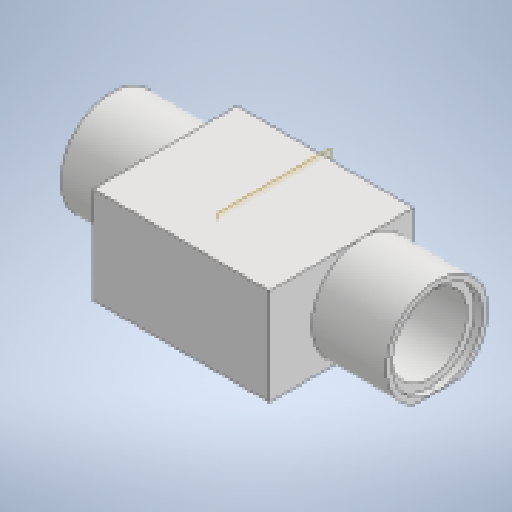
# Autodesk Inventor part: motors_mount
Saved by Autodesk Inventor 2023 (Build 270158000, 158)
## iProperties
Created: 2025-01-11
Part Number: motors_mount
Material: Ogólny
Document SubType Name: Modeling
Designer: kamil
Density: 1 g/cm^3
Appearance: Domyślna
Author: kamil
Autodesk Inventor part; units mm, degrees
ref_plane "YZ Plane" through (0, 0, 0) normal (1, 0, 0) x (0, 1, 0)
ref_plane "XZ Plane" through (0, 0, 0) normal (0, 1, 0) x (-1, 0, 0)
ref_plane "XY Plane" through (0, 0, 0) normal (0, 0, 1) x (1, 0, 0)
sketch "Szkic1" plane through (0, 0, 0) normal (1, 0, 0) x (0, 1, 0)
  circle A0 centre (0, 0) radius 11
  dimension "d0" = 22
  constraints: 1 centre point, 1 coincident
  measures "d0" diameter of A0
extrude "Wyciągnięcie proste1" add sketch "Szkic1" along normal blind 70
sketch "Szkic2" plane through (70, 0, 0) normal (1, 0, 0) x (0, 0, -1)
  circle A0 centre (0, 0) radius 11 projected
  circle A1 centre (0, 0) radius 9.75
  dimension "d3" = 19.5
  constraints: 1 centre point, 1 coincident
  measures "d3" diameter of A1
extrude "Wyciągnięcie proste2" cut sketch "Szkic2" against normal blind 1.6 contours A1
sketch "Szkic3" plane through (68.4, 0, 0) normal (1, 0, 0) x (0, 0, -1)
  circle A0 centre (0, 0) radius 9.75 projected
  circle A1 centre (0, 0) radius 8.15
  dimension "d6" = 16.3
  constraints: 1 centre point, 1 coincident
  measures "d6" diameter of A1
extrude "Wyciągnięcie proste3" cut sketch "Szkic3" against normal blind 31 contours A1
ref_plane "Płaszczyzna konstrukcyjna1" through (35, 0, 0) normal (1, 0, 0) x (0, 0, -1)
mirror "Odbij1" about plane through (35, 0, 0) normal (1, 0, 0) of "Wyciągnięcie proste3", "Wyciągnięcie proste2"
sketch "Szkic4" plane through (70, 0, 0) normal (1, 0, 0) x (0, 0, -1)
  circle A0 centre (0, 0) radius 11 projected
  line L0 (-20, 11) -> (11, 11)
  line L1 (11, 11) -> (11, -11)
  line L2 (11, -11) -> (-20, -11)
  line L3 (-20, -11) -> (-20, 11)
  point P0 (0, -11)
  point P1 (0, 11)
  dimension "d9" = 20
  constraints: 8 end point, 3 tangent, 2 parallel, 1 horizontal, 1 perpendicular
  measures "d9" distance from line of L3 point (0, 0)
extrude "Wyciągnięcie proste4" add sketch "Szkic4" against normal up to surface (70 mm away) contours A0 L2 L3 L0
sketch "Szkic5" plane through (70, 11, 20) normal (0, 1, 0) x (1, 0, 0)
  line L0 (-70, 0) -> (-70, 20) projected
  line L1 (-70, 31) -> (0, 31) projected
  line L2 (-37.4, 28.15) -> (-37.4, 11.85) projected
  line L3 (-68.4, 11.85) -> (-68.4, 28.15) projected
  line L4 (-37.4, 28.15) -> (-37.4, 11.85) projected
  line L5 (-37.4, 28.15) -> (-68.4, 28.15)
  line L6 (-37.4, 28.15) -> (-68.4, 28.15) projected
  line L7 (-68.4, 11.85) -> (-37.4, 11.85)
  line L8 (-70, 10.25) -> (-70, 29.75) projected
  line L9 (0, 0) -> (-70, 0) projected
  line L10 (-70, 0) -> (-54, 0)
  line L11 (-54, 0) -> (-54, 9)
  line L12 (-54, 9) -> (-70, 9)
  line L13 (-70, 9) -> (-70, 0)
  line L14 (0, 0) -> (-16, 0)
  line L15 (-16, 0) -> (-16, 9)
  line L16 (-16, 9) -> (0, 9)
  line L17 (0, 9) -> (0, 0)
  point P0 (-16, 0)
  dimension "d12" = 16
  dimension "d13" = 2.85
  dimension "d14" = 16
  constraints: 20 end point, 5 equal length, 3 perpendicular, 2 horizontal
  measures "d12" distance of L12.end L11.end
  measures "d13" distance between parallel lines of L7 L12
  measures "d14" distance of L15.end L16.end
extrude "Wyciągnięcie proste5" cut sketch "Szkic5" along normal through all both and the other way through all contours L0 L12 L11 L9 | L9 L15 L16 L17
sketch "Szkic6" plane through (0, 0, 0) normal (-1, 0, 0) x (0, 0, 1)
  arc A0 (0, 11) -> (0, -11) centre (0, 0) ccw projected
  circle A1 centre (0, 0) radius 11
  line L0 (11, -11) -> (11, 11) projected
  line L1 (11, 11) -> (0, 11) projected
  arc A2 (0, 11) -> (0, -11) centre (0, 0) ccw projected
  line L2 (0, -11) -> (11, -11) projected
  circle A3 centre (0, 0) radius 9.75 projected
  point P0 (0, -11)
  point P1 (11, 0)
  constraints: 1 coincident, 3 other
extrude "Wyciągnięcie proste6" cut sketch "Szkic6" against normal up to surface (16 mm away) contours L1 L0 A1 | A1 L0 L2
mirror "Odbij2" about plane through (35, 0, 0) normal (1, 0, 0) of "Wyciągnięcie proste6"
sketch "Szkic7" plane through (70, 0, 0) normal (1, 0, 0) x (0, 0, -1)
  line L0 (0, -11) -> (-20, -11) projected
  circle A0 centre (0, 0) radius 9.75 projected
  line L1 (-20, -11) -> (0, -11) projected
  line L2 (-20, -11) -> (9.75, -11)
  line L3 (9.75, -11) -> (9.75, -9.75)
  line L4 (9.75, -9.75) -> (-20, -9.75)
  line L5 (-20, -9.75) -> (-20, -11)
  constraints: 8 end point, 2 parallel, 2 tangent, 1 horizontal, 1 perpendicular
extrude "Wyciągnięcie proste7" cut sketch "Szkic7" against normal through all contours L0 L5 L4 L3 L2
sketch "Szkic8" plane through (54, 11, 20) normal (1, 0, 0) x (0, 0, -1)
  arc A0 (25.0929, -20.75) -> (14.9071, -20.75) centre (20, -11) ccw projected
  line L0 (0, -20.75) -> (14.9071, -20.75) projected
  line L1 (20, 0) -> (0, 0) projected
  line L2 (20, 0) -> (31, 0)
  line L3 (31, 0) -> (31, -20.75)
  line L4 (31, -20.75) -> (20, -20.75)
  line L5 (20, -20.75) -> (20, 0)
  point P0 (31, -11)
  constraints: 8 end point, 2 parallel, 1 collinear, 1 horizontal, 1 perpendicular, 1 tangent
extrude "Wyciągnięcie proste8" add sketch "Szkic8" against normal up to surface (38 mm away) contours A0 L3 L4 | A0 L2 L3
sketch "Szkic9" plane through (16, 11, 20) normal (0, 0, 1) x (1, 0, 0)
  line L0 (0, -20.75) -> (38, -20.75) projected
  line L1 (38, -20.75) -> (38, 0) projected
  line L2 (38, 0) -> (0, 0) projected
  line L3 (0, 0) -> (0, -20.75) projected
  point P0 (-16, -11)
extrude "Wyciągnięcie proste9" cut sketch "Szkic9" against normal blind 3
sketch "Szkic10" plane through (54, 11, 0) normal (0, 1, 0) x (1, 0, 0)
  line L0 (-38, -17) -> (0, -17) projected
  line L1 (0, -17) -> (0, 0) projected
  line L2 (0, 11) -> (0, 0) projected
  line L3 (0, 11) -> (-38, 11) projected
  line L4 (-38, 0) -> (-38, 11) projected
  line L5 (-38, 0) -> (-38, -17) projected
  point P0 (-54, 0)
  point P1 (-10, -13)
  point P2 (-28, -13)
  point P3 (-19, 5.5)
  point P4 (-19, 11)
  dimension "d26" = 10
  dimension "d27" = 4
  dimension "d28" = 10
  dimension "d29" = 4
  dimension "d30" = 5.5
  constraints: 1 midpoint, 1 vertical alignment
  measures "d26" distance from line of L1 point (-10, -13)
  measures "d27" distance from line of L0 point (-10, -13)
  measures "d28" distance from line of L5 point (-28, -13)
  measures "d29" distance from line of point (-28, -13) L0
  measures "d30" distance from line of L3 point (-19, 5.5)
hole "Otwór1" at (44, 11, 13) at (26, 11, 13) at (35, 11, -5.5) direction (0, -1, 0) diameter 3.4 end through all
sketch "Szkic11" plane through (54, 11, 0) normal (0, 1, 0) x (1, 0, 0)
  circle A0 centre (-19, 5.5) radius 1.7 projected
  circle A1 centre (-19, 5.5) radius 2.8
  line L0 (0, 11) -> (-38, 11) projected
  line L1 (0, 11) -> (-38, 11) projected
  line L2 (-21.8, 5.5) -> (-16.2, 5.5)
  line L3 (-16.2, 5.5) -> (-16.2, 11)
  line L4 (-16.2, 11) -> (-21.8, 11)
  line L5 (-21.8, 11) -> (-21.8, 5.5)
  point P0 (-54, 0)
  dimension "d38" = 1.1
  constraints: 8 end point, 2 parallel, 2 vertical, 1 horizontal, 1 perpendicular, 1 point on line, 3 other
extrude "Wyciągnięcie proste10" add sketch "Szkic11" against normal up to surface (20.75 mm away) contours L2 A1 A0 | A0 L2 A1 | A1 L5 L0 L3
chamfer "Faza1" distance 1 angle 45 1 edges at (35, -9.75, -11)
sketch "Szkic12" plane through (68.4, 0, 0) normal (1, 0, 0) x (0, 0, -1)
  circle A0 centre (0, 0) radius 9.75 projected
  line L0 (0, 0) -> (-6.2672, 7.4689)
  circle A1 centre (0, 0) radius 9.75 projected
  line L1 (0, 0) -> (9.75, 0) construction
  line L2 (-6.2672, 7.4689) -> (-5.0415, 8.4974)
  line L3 (-5.0415, 8.4974) -> (1.6116, 0.5686)
  line L4 (-6.2672, 7.4689) -> (-7.4929, 6.4405)
  line L5 (-7.4929, 6.4405) -> (-3.3968, 1.559)
  circle A2 centre (0, 0) radius 8.15 projected
  point P0 (0, -9.75)
  point P1 (-6.3624, 5.0933)
  point P2 (-3.9111, 7.1502)
  point P3 (-4.9565, 8.3961)
  point P4 (-7.4079, 6.3392)
  dimension "d44" = 130
  dimension "d45" = 1.6
  dimension "d46" = 1.6
  constraints: 12 end point, 1 collinear, 1 equal length, 1 horizontal, 1 parallel, 1 perpendicular, 1 point on circle, 1 tangent, 2 other
  measures "d44" angle of L1 L0
  measures "d45" distance of L0.end L2.end
  measures "d46" distance between parallel lines of L0 L5
extrude "Wyciągnięcie proste11" cut sketch "Szkic12" against normal up to surface (31 mm away) contours L3 A2 L0 A0 | A0 L0 A2 L5
sketch "Szkic13" plane through (16, 11, 17) normal (0, 0, 1) x (1, 0, 0)
  line L0 (38, 0) -> (38, -20.75) projected
  line L1 (0, 0) -> (38, 0) projected
  line L2 (0, -20.75) -> (0, 0) projected
  line L3 (38, -20.75) -> (0, -20.75) projected
  line L4 (21.4, -2.6039) -> (24.4, -2.6039)
  line L5 (24.4, -2.6039) -> (24.4, -4.6608)
  line L6 (24.4, -4.6608) -> (21.4, -4.6608)
  line L7 (21.4, -4.6608) -> (21.4, -2.6039)
  point P0 (-16, -11)
  dimension "d49" = 3
  constraints: 8 end point, 2 parallel, 1 coincident, 1 horizontal, 1 perpendicular
  measures "d49" distance of L5.end L6.end
extrude "Wyciągnięcie proste12" cut sketch "Szkic13" against normal up to surface (12.0435 mm away) contours L4 L5 L6 L7
sketch "Szkic14" plane through (37.4, 0, 0) normal (1, 0, 0) x (0, 0, -1)
  line L0 (-6.3624, 5.0933) -> (-7.4079, 6.3392) projected
  arc A0 (-6.3624, 5.0933) -> (4.0578, -7.068) centre (0, 0) ccw projected
  line L1 (4.0578, -7.068) -> (4.0578, 7.068) projected
  arc A1 (4.0578, 7.068) -> (-3.9111, 7.1502) centre (0, 0) ccw projected
  line L2 (-4.9565, 8.3961) -> (-3.9111, 7.1502) projected
  line L3 (-17, 8.3961) -> (-4.9565, 8.3961) projected
  line L4 (-17, 6.3392) -> (-17, 8.3961) projected
  line L5 (-17, 6.3392) -> (-7.4079, 6.3392) projected
  circle A2 centre (-7.9579, 5.0933) radius 0.2358
  arc A3 (-4.9565, 8.3961) -> (-7.4079, 6.3392) centre (0, 0) ccw projected
  line L6 (-6.3624, 5.0933) -> (-7.2006, 5.8335) construction
  line L7 (-7.2006, 5.8335) -> (-10.2204, 6.3392) construction
  spline S0 degree 2 poles (-6.3624, 5.0933) (-7.2006, 5.8335) (-10.2204, 6.3392) knots 1 1 1 2 2 2
  constraints: 1 centre point, 1 point on line, 3 other
extrude "Wyciągnięcie proste13" cut sketch "Szkic14" along normal up to surface (3 mm away) contours S0 L5 L0
mirror "Odbij3" about plane through (35, 0, 0) normal (1, 0, 0) of "Wyciągnięcie proste13", "Wyciągnięcie proste12", "Wyciągnięcie proste11"
sketch "Szkic17" plane through (16, 11, 17) normal (0, 0, 1) x (1, 0, 0)
  line L0 (24.4, -4.6608) -> (21.4, -4.6608) projected
  line L1 (21.4, -4.6608) -> (21.4, -2.6039) projected
  line L2 (21.4, -4.6608) -> (24.4, -4.6608)
  line L3 (24.4, -4.6608) -> (24.4, -6.1608)
  line L4 (24.4, -6.1608) -> (21.4, -6.1608)
  line L5 (21.4, -6.1608) -> (21.4, -4.6608)
  point P0 (-16, -11)
  dimension "d62" = 1.5
  constraints: 8 end point, 2 parallel, 1 horizontal, 1 perpendicular, 1 vertical alignment
  measures "d62" distance of L2.end L3.end
extrude "Wyciągnięcie proste16" cut sketch "Szkic17" against normal blind 12
mirror "Odbij4" about plane through (35, 0, 0) normal (1, 0, 0) of "Wyciągnięcie proste16"
fillet "Zaokrąglenie4" radius 1 2 edges at (31.1, 4.8392, 6.5578) (38.9, 4.8392, 6.5578)
fillet "Zaokrąglenie5" radius 0.6 4 edges at (54.4, 5.0933, 6.3624) (52.9, 7.1502, 3.9111) (15.6, 5.0933, 6.3624) (17.1, 7.1502, 3.9111)
fillet "Zaokrąglenie6" radius 1 2 edges at (40.4, 7.4689, 6.2672) (29.6, 7.4689, 6.2672)
sketch "Szkic18" plane through (54, 11, 0) normal (0, 1, 0) x (1, 0, 0)
  circle A0 centre (-28, -13) radius 1.7 projected
  circle A1 centre (-10, -13) radius 1.7 projected
  circle A2 centre (-19, 5.5) radius 1.7 projected
  circle A3 centre (-28, -13) radius 2.9
  circle A4 centre (-10, -13) radius 2.9
  circle A5 centre (-19, 5.5) radius 2.9
  circle A6 centre (-28, -13) radius 1.7 projected
  line L0 (-29.6743, -15.9) -> (-31.3486, -13)
  line L1 (-31.3486, -13) -> (-29.6743, -10.1)
  line L2 (-29.6743, -10.1) -> (-26.3257, -10.1)
  line L3 (-26.3257, -10.1) -> (-24.6514, -13)
  line L4 (-24.6514, -13) -> (-26.3257, -15.9)
  line L5 (-26.3257, -15.9) -> (-29.6743, -15.9)
  circle A7 centre (-10, -13) radius 1.7 projected
  line L6 (-11.6743, -15.9) -> (-13.3486, -13)
  line L7 (-13.3486, -13) -> (-11.6743, -10.1)
  line L8 (-11.6743, -10.1) -> (-8.3257, -10.1)
  line L9 (-8.3257, -10.1) -> (-6.6514, -13)
  line L10 (-6.6514, -13) -> (-8.3257, -15.9)
  line L11 (-8.3257, -15.9) -> (-11.6743, -15.9)
  line L12 (-17.3323, 8.4038) -> (-15.6514, 5.5077)
  line L13 (-15.6514, 5.5077) -> (-17.319, 2.6039)
  line L14 (-17.319, 2.6039) -> (-20.6677, 2.5962)
  line L15 (-20.6677, 2.5962) -> (-22.3486, 5.4923)
  line L16 (-22.3486, 5.4923) -> (-20.681, 8.3961)
  line L17 (-20.681, 8.3961) -> (-17.3323, 8.4038)
  point P0 (-54, 0)
  point P1 (-28, -15.9)
  point P2 (-10, -15.9)
  point P3 (-19.0067, 8.4)
  dimension "d68" = 5.8
  dimension "d69" = 5.8
  dimension "d70" = 5.8
  constraints: 36 end point, 6 coincident, 3 midpoint, 2 point on line, 2 vertical alignment, 46 other
extrude "Wyciągnięcie proste17" cut sketch "Szkic18" against normal blind 6 contours A0 | A1 | A2 | A3 | A3 L3 L4 | A3 L2 L3 | L4 L5 A3 | A3 L1 L2 | L5 L0 A3 | A3 L0 L1 | A4 | A4 L9 L10 | A4 L8 L9 | L10 L11 A4 | A4 L7 L8 | L11 L6 A4 | A4 L6 L7 | A5 | A5 L12 L13 | A5 L17 L12 | L13 L14 A5 | A5 L16 L17 | L14 L15 A5 | A5 L15 L16
sketch "Szkic19" plane through (54, 11, 0) normal (0, 1, 0) x (1, 0, 0)
  circle A0 centre (-28, -13) radius 1.7 projected
  circle A1 centre (-10, -13) radius 1.7 projected
  circle A2 centre (-19, 5.5) radius 1.7 projected
  circle A3 centre (-28, -13) radius 1.7 projected
  circle A4 centre (-28, -13) radius 3.5
  circle A5 centre (-10, -13) radius 1.7 projected
  circle A6 centre (-10, -13) radius 3.5
  circle A7 centre (-19, 5.5) radius 3.5
  point P0 (-54, 0)
  dimension "d73" = 7
  dimension "d74" = 7
  dimension "d75" = 7
  constraints: 3 centre point, 3 coincident
  measures "d73" diameter of A4
  measures "d74" diameter of A6
  measures "d75" diameter of A7
extrude "Wyciągnięcie proste18" cut sketch "Szkic19" against normal blind 3 contours A0 | A1 | A2 | A4 | A6 | A7
sketch "Szkic20" plane through (16, 11, 17) normal (0, 0, 1) x (1, 0, 0)
  line L0 (-14.4, -19.15) -> (-14.4, -2.85) projected
  line L1 (0, -20.75) -> (0, 0) projected
  point P0 (-16, -11)
  point P1 (-14.4, -6.2745)
  point P2 (-14.4, -3.6401)
  point P3 (4, -11)
  point P4 (-14.4, -11)
  dimension "d78" = 4
  constraints: 1 horizontal alignment, 1 midpoint
  measures "d78" distance from line of point (4, -11) L1
hole "Otwór2" at (20, 0, 17) direction (0, 0, -1) diameter 3.4 depth 10 tip angle 118 counterbore diameter 6 counterbore depth 3
ref_plane "Płaszczyzna konstrukcyjna2" through (54, 0, 7) normal (0, 0, -1) x (-1, 0, 0)
sketch "Szkic21" plane through (54, 0, 7) normal (0, 0, -1) x (-1, 0, 0)
  circle A0 centre (34, 0) radius 1.7 projected
  circle A1 centre (34, 0) radius 2.95
  line L0 (36.95, -1.7032) -> (34, -3.4064)
  line L1 (34, -3.4064) -> (31.05, -1.7032)
  line L2 (31.05, -1.7032) -> (31.05, 1.7032)
  line L3 (31.05, 1.7032) -> (34, 3.4064)
  line L4 (34, 3.4064) -> (36.95, 1.7032)
  line L5 (36.95, 1.7032) -> (36.95, -1.7032)
  line L6 (38, -9.75) -> (38, 11) projected
  point P0 (54, 0)
  point P1 (36.95, 0)
  dimension "d87" = 5.9
  constraints: 12 end point, 2 coincident, 1 horizontal alignment, 1 midpoint, 1 parallel, 16 other
extrude "Wyciągnięcie proste19" cut sketch "Szkic21" against normal blind 4.5 contours A0 | A1 | L5 L0 A1 | A1 L4 L5 | A1 L3 L4 | L0 L1 A1 | A1 L2 L3 | L1 L2 A1
mirror "Odbij5" about plane through (35, 0, 0) normal (1, 0, 0) of "Wyciągnięcie proste19", "Otwór2"
